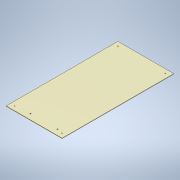
# Autodesk Inventor part: top_bottom_layer_3mm
Saved by Autodesk Inventor 2021 (Build 250183000, 183)
## iProperties
Created: 2021-01-27
Part Number: top_bottom_layer_3mm
Material: Acrylic
Document SubType Name: Modeling
Designer: abij996
Density: 1.188 g/cm^3
Appearance: Smooth - Ash
Author: abij996
Autodesk Inventor part; units mm, degrees
ref_plane "YZ Plane" through (0, 0, 0) normal (1, 0, 0) x (0, 1, 0)
ref_plane "XZ Plane" through (0, 0, 0) normal (0, 1, 0) x (-1, 0, 0)
ref_plane "XY Plane" through (0, 0, 0) normal (0, 0, 1) x (1, 0, 0)
sketch "Sketch2" plane through (0, 0, 0) normal (0, 1, 0) x (-1, 0, 0)
  line L0 (238.7833, 365.019) -> (-161.2167, 365.019)
  line L1 (-161.2167, 365.019) -> (-161.2167, -434.981)
  line L2 (-161.2167, -434.981) -> (238.7833, -434.981)
  line L3 (238.7833, -434.981) -> (238.7833, 365.019)
  circle A0 centre (-131.2167, 335.019) radius 3
  circle A1 centre (208.7833, -404.981) radius 3
  circle A2 centre (208.7833, 335.019) radius 3
  circle A3 centre (-131.2167, -404.981) radius 3
  circle A4 centre (104.0333, 326.519) radius 4
  circle A5 centre (-89.9667, 326.519) radius 4
  point P0 (0, 0)
  dimension "d46" = 800
  dimension "d47" = 400
  dimension "d50" = 6
  dimension "d51" = 6
  dimension "d52" = 30
  dimension "d53" = 30
  dimension "d54" = 30
  dimension "d55" = 30
  dimension "d58" = 6
  dimension "d59" = 6
  dimension "d60" = 30
  dimension "d61" = 30
  dimension "d62" = 30
  dimension "d63" = 30
  dimension "d66" = 8
  dimension "d67" = 38.5
  dimension "d68" = 134.75
  dimension "d69" = 8
  dimension "d70" = 71.25
  dimension "d71" = 38.5
  constraints: 8 end point, 6 centre point, 2 parallel, 1 horizontal, 1 perpendicular
  measures "d46" distance of L2.end L0.start
  measures "d47" distance of L0.start L0.end
  measures "d50" diameter of A0
  measures "d51" diameter of A1
  measures "d52" distance from line of L3 A1.centre
  measures "d53" distance from line of L2 A1.centre
  measures "d54" distance from line of L1 A0.centre
  measures "d55" distance from line of L0 A0.centre
  measures "d58" diameter of A2
  measures "d59" diameter of A3
  measures "d60" distance from line of L3 A2.centre
  measures "d61" distance from line of L0 A2.centre
  measures "d62" distance from line of L1 A3.centre
  measures "d63" distance from line of L2 A3.centre
  measures "d66" diameter of A4
  measures "d67" distance from line of L0 A4.centre
  measures "d68" distance from line of L3 A4.centre
  measures "d69" diameter of A5
  measures "d70" distance from line of L1 A5.centre
  measures "d71" distance from line of L0 A5.centre
extrude "Extrusion6" add sketch "Sketch2" along normal blind 3
body "Solid6"
